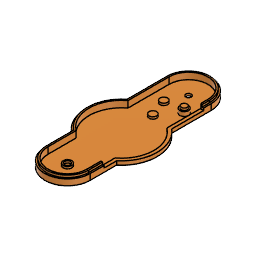
UpperHousing (Autodesk Fusion 360 design; units mm, degrees)
part number: 2026-06-04-23-22-25-644
Autodesk Fusion 360 part; units mm, degrees
sketch "Sketch1" plane through (0, 0, 0) normal (0, 0, 1) x (1, 0, 0)
  circle A0 centre (-2.9141, 22.4848) radius 1.25
  line L0 (-9, 12) -> (-9, 31)
  arc A1 (9, -12) -> (9, 12) centre (0, 0) ccw
  arc A2 (-10.5, -25) -> (10.5, -25) centre (0, -25) ccw
  line L1 (0, 0) -> (0, 12) construction
  circle A3 centre (0, 0) radius 3
  arc A4 (9, 31) -> (-9, 31) centre (0, 31) ccw
  arc A5 (10.5, -12.7279) -> (10.5, 12.7279) centre (0, 0) ccw
  circle A6 centre (0, 31) radius 1.25
  line L2 (-10.5, -25) -> (-10.5, -12.7279)
  arc A7 (-9, 12) -> (-9, -12) centre (0, 0) ccw
  line L3 (9, -25) -> (9, -12)
  circle A8 centre (0, 0) radius 12 construction
  circle A9 centre (-2.9141, 22.4848) radius 2.5 construction
  line L4 (10.5, -25) -> (10.5, -12.7279)
  circle A10 centre (0, 14.5) radius 2.5 construction
  arc A11 (-9, -25) -> (9, -25) centre (0, -25) ccw
  line L5 (-9, -25) -> (-9, -12)
  line L6 (0, -25) -> (0, 0) construction
  arc A12 (10.5, 31) -> (-10.5, 31) centre (0, 31) ccw
  circle A13 centre (0, 14.5) radius 6 construction
  line L7 (10.5, 12.7279) -> (10.5, 31)
  line L8 (-10.5, 12.7279) -> (-10.5, 31)
  circle A14 centre (0, 14.5) radius 1.25
  line L9 (0, 14.5) -> (0, 12) construction
  arc A15 (-10.5, 12.7279) -> (-10.5, -12.7279) centre (0, 0) ccw
  line L10 (-9, 21.5) -> (-10.5, 21.5) construction
  line L11 (-6, 23) -> (-9, 23) construction
  circle A16 centre (0, 31) radius 4.5 construction
  line L12 (9, 12) -> (9, 31)
  circle A17 centre (-2.9141, 22.4848) radius 4.5 construction
  line L13 (9, 21.5) -> (10.5, 21.5) construction
  line L14 (9, 27.5) -> (10.5, 27.5)
  line L15 (9, 23) -> (10.5, 23) construction
  line L16 (9, 23) -> (6, 23) construction
  circle A18 centre (6, 23) radius 2
  arc A19 (9.75, 31) -> (-9.75, 31) centre (0, 31) ccw
  line L17 (-9.75, 12.3693) -> (-9.75, 31)
  arc A20 (-9.75, 12.3693) -> (-9.75, -12.3693) centre (0, 0) ccw
  line L18 (-9.75, -25) -> (-9.75, -12.3693)
  arc A21 (-9.75, -25) -> (9.75, -25) centre (0, -25) ccw
  line L19 (9.75, -25) -> (9.75, -18.5)
  line L20 (9.75, 27.5) -> (9.75, 31)
  line L21 (9, -18.5) -> (10.5, -18.5)
  circle A22 centre (6, 23) radius 1.375
  circle A23 centre (0, 0) radius 2
  circle A24 centre (0, -25) radius 2
  circle A25 centre (0, -25) radius 1.375
  circle A26 centre (0, 14.5) radius 1.75
  circle A27 centre (-2.9141, 22.4848) radius 1.75
  dimension "d1" = 1.5
  dimension "d3" = 56
  dimension "d4" = 30
  dimension "d5" = 18
  dimension "d6" = 18
  dimension "d7" = 6
  dimension "d8" = 24
  dimension "d9" = 25
  dimension "d10" = 12
  dimension "d11" = 5
  dimension "d12" = 9
  dimension "d13" = 5
  dimension "d14" = 9
  dimension "d15" = 15
  dimension "d16" = 2.5
  dimension "d17" = 2.5
  dimension "d18" = 2.5
  dimension "d19" = 3
  dimension "d20" = 8
  dimension "d28" = 6
  dimension "d29" = 8
  dimension "d30" = 3
  dimension "d31" = 4
  dimension "d33" = 3.5
  dimension "d34" = 15.75
  dimension "d35" = 2.75
  dimension "d36" = 4
  dimension "d37" = 2.75
  dimension "d38" = 4
  dimension "d47" = 3.5
  dimension "d48" = 3.5
  constraint coincident A1.centre L1.start
  constraint tangent L0 A4
  constraint tangent A4 L12
  constraint concentric A7 A8
  constraint parallel L3 L5
  constraint vertical L5
  constraint coincident A2.centre A11.centre
  constraint parallel L3 L6
  constraint parallel L1 L6
  constraint concentric A10 A13
  constraint concentric A4 A16
  constraint concentric A9 A17
  constraint tangent A16 A17
  constraint coincident A10.centre A13.centre
  constraint coincident L1.end A10
  constraint vertical L9
  constraint coincident L1.end A8
  constraint collinear L0 L5
  constraint collinear L3 L12
  constraint concentric A1 A7
  constraint concentric A13 A14
  constraint concentric A0 A9
  constraint concentric A6 A16
  constraint horizontal L11
  constraint coincident L11.end L0
  constraint midpoint L10.start L0
  constraint coincident L10.end L8
  constraint perpendicular L8 L10
  constraint tangent A9 A13
  constraint midpoint L12 L13.start
  constraint coincident L7 L13.end
  constraint perpendicular L7 L13
  constraint coincident L12 L14.start
  constraint coincident L7 L14.end
  constraint perpendicular L7 L14
  constraint coincident L12 L15.start
  constraint coincident L7 L15.end
  constraint perpendicular L7 L15
  constraint perpendicular L12 L16
  constraint coincident L16.end A18.centre
  constraint concentric A4 A19
  constraint concentric A7 A20
  constraint concentric A11 A21
  constraint tangent A19 L20
  constraint tangent A19 L17
  constraint tangent L18 A21
  constraint coincident L14 L20.start
  constraint midpoint L3 L21.start
  constraint coincident L4 L21.end
  constraint perpendicular L4 L21
  constraint coincident L21 L19.end
  constraint concentric A18 A22
  constraint concentric A7 A23
  constraint concentric A11 A24
  constraint concentric A24 A25
  constraint concentric A13 A26
  constraint concentric A0 A27
  measures "d3" distance of A2.centre A4.centre
  measures "d4" diameter of A7
  measures "d5" diameter of A4
  measures "d6" diameter of A11
  measures "d7" diameter of A3
  measures "d8" diameter of A8
  measures "d9" distance of A1.centre A2.centre
  measures "d10" diameter of A13
  measures "d11" diameter of A10
  measures "d12" diameter of A16
  measures "d13" diameter of A9
  measures "d14" diameter of A17
  measures "d15" radius of A1
  measures "d16" diameter of A14
  measures "d17" diameter of A0
  measures "d18" diameter of A6
  measures "d19" distance of L11.start L11.end
  measures "d20" distance of A4.centre L11
  measures "d28" distance of L13 L14
  measures "d29" distance of A4.centre L15
  measures "d30" distance of L15.start L16.end
  measures "d31" diameter of A18
  measures "d33" distance of A19.start L20.start
  measures "d34" radius of A20
  measures "d35" diameter of A22
  measures "d36" diameter of A23
  measures "d37" diameter of A25
  measures "d38" diameter of A24
  measures "d47" diameter of A26
  measures "d48" diameter of A27
extrude "Extrude1" add sketch "Sketch1" along normal blind 1 contours L0 A1 A4 A7 L3 A11 L5 L12 | A1 A5 L3 L4 L7 L12 L14 L21 | A26 | A27
extrude "Extrude4" add sketch "Sketch1" along normal blind 2 contours A1 A5 L3 L4 L7 L12 L14 L21
extrude "Extrude5" add sketch "Sketch1" along normal blind 1.95 contours A0 | A14 | A26 | A27
extrude "Extrude6" add sketch "Sketch1" along normal blind 2.95 contours A18 | A22
extrude "Extrude7" add sketch "Sketch1" along normal blind 3.95 contours A22
extrude "Extrude8" add sketch "Sketch1" along normal blind 1 contours A3 | A23
extrude "Extrude9" add sketch "Sketch1" along normal blind 1.95 contours A24 | A25
extrude "Extrude10" cut sketch "Sketch1" along normal blind 1.5 from surface at 1 contours A25
extrude "Extrude2" add sketch "Sketch1" along normal blind 3 contours A2 L2 L4 A12 L7 L8 A15 L14 A19 L17 A20 L18 A21 L19 L20 L21
extrude "Extrude3" add sketch "Sketch1" along normal blind 4 contours L0 A4 A7 L3 A11 L5 L12 L14 A19 L17 A20 L18 A21 L19 L20 L21
fillet "Fillet1" radius 0.25 9 edges at (9, 27.5, 3) (-10.5, -18.864, 0) (0, -35.5, 0) (10.5, -18.864, 0) (16.5, 0, 0) (10.5, 21.864, 0) (0, 41.5, 0) (-10.5, 21.8639, 0) (-16.5, 0, 0)
equation "d6 = d5"
